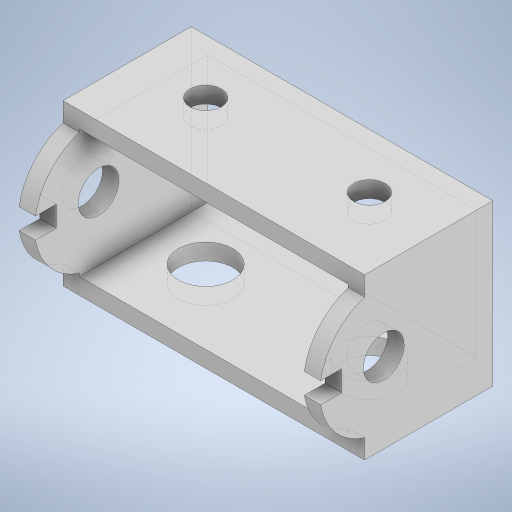
# Autodesk Inventor part: Xgantry_CableChain_bottom_connector
Saved by Autodesk Inventor 2023 (Build 270158000, 158)
## iProperties
Created: 2023-01-07
Part Number: Xgantry_CableChain_bottom_connector
Material: Generic
Document SubType Name: Modeling
Designer: a laptop
Density: 1 g/cm^3
Appearance: Default
Author: a laptop
Autodesk Inventor part; units mm, degrees
ref_plane "YZ Plane" through (0, 0, 0) normal (1, 0, 0) x (0, 1, 0)
ref_plane "XZ Plane" through (0, 0, 0) normal (0, 1, 0) x (-1, 0, 0)
ref_plane "XY Plane" through (0, 0, 0) normal (0, 0, 1) x (1, 0, 0)
sketch "Sketch1" plane through (0, 0, 0) normal (1, 0, 0) x (0, 1, 0)
  arc A0 (-1.9, 11.5447) -> (-11.7, 0) centre (0, 0) ccw
  line L0 (1.9, 11.5447) -> (1.9, 7.75)
  line L1 (1.9, 7.75) -> (-1.9, 7.75)
  line L2 (-1.9, 7.75) -> (-1.9, 11.5447)
  line L3 (0, 7.75) -> (0, 0) construction
  arc A1 (1.9, 11.5447) -> (-1.9, 11.5447) centre (0, 0) ccw construction
  circle A2 centre (0, 0) radius 3.75
  line L4 (11.7, 0) -> (11.7, -20)
  line L5 (11.7, -20) -> (-11.7, -20)
  line L6 (-11.7, -20) -> (-11.7, 0)
  arc A3 (11.7, 0) -> (1.9, 11.5447) centre (0, 0) ccw
  arc A4 (-11.7, 0) -> (11.7, 0) centre (0, 0) ccw construction
  dimension "d0" = 23.4
  dimension "d1" = 3.8
  dimension "d2" = 7.75
  dimension "d3" = 7.5
  dimension "d9" = 20
  constraints: 14 end point, 9 point on circle, 5 centre point, 3 tangent, 3 vertical, 2 coincident, 2 parallel, 2 perpendicular, 1 horizontal alignment, 1 midpoint
  measures "d0" diameter of A0
  measures "d1" distance of L0.end L1.end
  measures "d2" distance from line of point (0, 0) L1
  measures "d3" diameter of A2
  measures "d9" distance from line of L5 point (0, 0)
extrude "Extrusion1" add sketch "Sketch1" along normal blind 3
pattern_linear "Rectangular Pattern1" count 2 spacing 52.25 along (-1, 0, 0) of "Extrusion1"
sketch "Sketch3" plane through (0, -11.7, -20) normal (0, -1, 0) x (1, 0, 0)
  line L0 (-52.25, 0) -> (-49.25, 0) projected
  line L1 (-52.25, 0) -> (3, 0)
  line L2 (3, 0) -> (3, 23.5)
  line L3 (3, 23.5) -> (-52.25, 23.5)
  line L4 (-52.25, 23.5) -> (-52.25, 0)
  point P0 (0, 20)
  dimension "d12" = 3.5
  constraints: 8 end point, 2 parallel, 1 coincident, 1 horizontal, 1 perpendicular
  measures "d12" distance from line of point (0, 20) L3
extrude "Extrusion3" add sketch "Sketch3" along normal blind 3
sketch "Sketch4" plane through (0, -11.7, -20) normal (0, 1, 0) x (1, 0, 0)
  line L0 (-49.25, -31.5447) -> (-49.25, -20) construction
  line L1 (-49.25, -20) -> (-52.25, -20)
  line L2 (-52.25, -20) -> (-52.25, -23.5)
  line L3 (-52.25, -23.5) -> (-49.25, -23.5)
  line L4 (-49.25, -23.5) -> (-49.25, -20)
  line L5 (0, -20) -> (0, 0) construction
  line L6 (3, -23.5) -> (-52.25, -23.5) construction
  line L7 (0, -20) -> (3, -20)
  line L8 (3, -20) -> (3, -23.5)
  line L9 (3, -23.5) -> (0, -23.5)
  line L10 (0, -23.5) -> (0, -20)
  constraints: 16 end point, 4 parallel, 2 horizontal, 2 perpendicular
extrude "Extrusion4" add sketch "Sketch4" along normal up to surface
mirror "Mirror1" about plane through (0, 0, 0) normal (0, 1, 0) of "Extrusion3", "Extrusion4"
sketch "Sketch9" plane through (-52.25, 14.7, -20) normal (0, 1, 0) x (1, 0, 0)
  circle A0 centre (12.625, -10) radius 2.8813
  circle A1 centre (42.625, -10) radius 2.8813
  line L0 (12.625, -10) -> (42.625, -10) construction
  line L1 (27.625, -10) -> (27.625, 0) construction
  line L2 (3, 0) -> (52.25, 0) construction
  point P0 (52.25, -20)
  dimension "d30" = 5.7625
  dimension "d31" = 30
  dimension "d32" = 10
  constraints: 4 end point, 2 centre point, 2 midpoint, 1 equal radius, 1 horizontal, 1 perpendicular
  measures "d30" diameter of A0
  measures "d31" distance of L0.start L0.end
  measures "d32" distance of L1.start L1.end
extrude "Extrusion9" cut sketch "Sketch9" against normal up to surface (3 mm away)
sketch "Sketch10" plane through (0, -14.7, -20) normal (0, -1, 0) x (1, 0, 0)
  circle A0 centre (-9.625, 10) radius 5
  circle A1 centre (-39.625, 10) radius 5
  circle A2 centre (-39.625, 10) radius 2.8813 construction
  circle A3 centre (-9.625, 10) radius 2.8813 construction
  point P0 (0, 20)
  dimension "d35" = 10
  constraints: 2 centre point, 2 concentric, 1 equal radius
  measures "d35" diameter of A1
extrude "Extrusion10" cut sketch "Sketch10" against normal up to surface (3 mm away)
body "Solid1"
